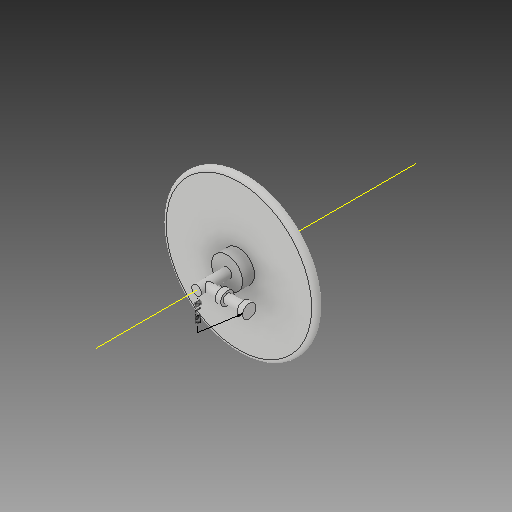
# Autodesk Inventor part: pizza wheel
Saved by Autodesk Inventor 2018 (Build 220112000, 112)
## iProperties
Created: 2018-02-16
Part Number: pizza wheel
Material: Generic
Document SubType Name: Modeling
Designer: allenr20
Density: 1 g/cm^3
Appearance: Default
Mass: 4991.4 g
Surface Area: 4238.99 cm^2
Volume: 4991.4 cm^3
Author: allenr20
Autodesk Inventor part; units mm, degrees
ref_plane "YZ Plane" through (0, 0, 0) normal (1, 0, 0) x (0, 1, 0)
ref_plane "XZ Plane" through (0, 0, 0) normal (0, 1, 0) x (-1, 0, 0)
ref_plane "XY Plane" through (0, 0, 0) normal (0, 0, 1) x (1, 0, 0)
sketch "Sketch1" plane through (0, 0, 0) normal (0, 0, 1) x (1, 0, 0)
  circle A0 centre (0, 0) radius 203.2
  circle A1 centre (0, 0) radius 241.3
  dimension "d0" = 406.4
  dimension "d1" = 38.1
  constraints: 2 centre point, 1 coincident
  measures "d0" diameter of A0
  measures "d1" radial gap between concentric circles of A0 A1
extrude "Extrusion1" add sketch "Sketch1" along normal blind 25.4 contours A0 | A1
fillet "Fillet1" radius 12.7 2 edges at (-241.3, 0, 25.4) (-241.3, 0, 0)
sketch "Sketch2" plane through (0, 0, 25.4) normal (0, 0, 1) x (1, 0, 0)
  circle A0 centre (0, 0) radius 48.9585
  dimension "d5" = 97.917
  constraints: 1 centre point, 1 coincident
  measures "d5" diameter of A0
extrude "Extrusion2" add sketch "Sketch2" along normal blind 37.211
sketch "Sketch3" plane through (0, 0, 62.611) normal (0, 0, 1) x (1, 0, 0)
  circle A0 centre (0, 0) radius 14.9225
  dimension "d8" = 29.845
  constraints: 1 centre point, 1 coincident
  measures "d8" diameter of A0
extrude "Extrusion3" add sketch "Sketch3" along normal blind 95.6056
sketch "Sketch5" plane through (0, 0, 0) normal (1, 0, 0) x (0, 1, 0)
  circle A0 centre (0, 131.7371) radius 13.6525
  line L0 (14.9225, 158.2166) -> (-14.9225, 158.2166) projected
  point P0 (0, 0)
  dimension "d11" = 27.305
  dimension "d12" = 26.4795
  constraints: 1 centre point
  measures "d11" diameter of A0
  measures "d12" distance from line of L0 A0.centre
extrude "Extrusion4" add sketch "Sketch5" along normal blind 133.8072
sketch "Sketch6" plane through (133.8072, 0, 131.7371) normal (1, 0, 0) x (0, 0, -1)
  circle A0 centre (0, 0) radius 13.6525 projected
  circle A1 centre (0, 0) radius 21.209
  point P0 (131.7371, 0)
  dimension "d15" = 42.418
  constraints: 1 centre point, 1 coincident
  measures "d15" diameter of A1
extrude "Extrusion5" add sketch "Sketch6" against normal blind 80.4672
sketch "Sketch8" plane through (133.8072, 0, 131.7371) normal (1, 0, 0) x (0, 0, -1)
  circle A0 centre (0, 0) radius 21.209
  point P0 (131.7371, 0)
  constraints: 1 centre point
extrude "Extrusion6" cut sketch "Sketch8" against normal blind 63.5
sketch "Sketch9" plane through (70.3072, 0, 131.7371) normal (1, 0, 0) x (0, 0, -1)
  circle A0 centre (0, 0) radius 13.6525 projected
  circle A1 centre (0, 0) radius 13.6525
  point P0 (131.7371, 0)
  constraints: 1 centre point, 1 coincident
extrude "Extrusion7" add sketch "Sketch9" along normal blind 51.6636
sketch "Sketch10" plane through (121.9708, 0, 131.7371) normal (1, 0, 0) x (0, 0, -1)
  circle A0 centre (0, 0) radius 21.209
  point P0 (131.7371, 0)
  constraints: 1 centre point
extrude "Extrusion8" add sketch "Sketch10" along normal blind 17.018
body "Solid1"
